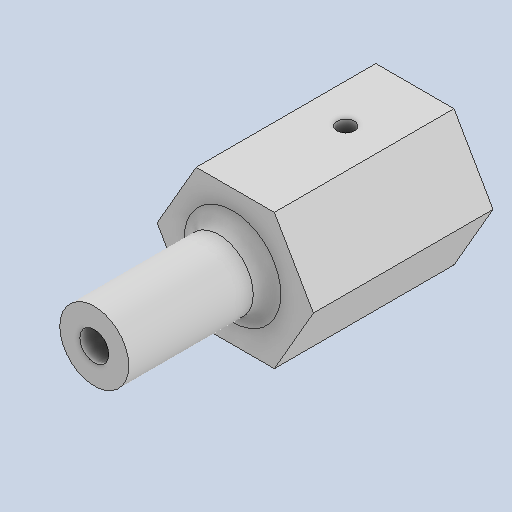
# Autodesk Inventor part: Acople_Motor
Saved by Autodesk Inventor 2022 (Build 260153000, 153)
## iProperties
Created: 2022-02-22
Part Number: Acople_Motor
Material: Generic
Document SubType Name: Modeling
Designer: katha
Density: 1 g/cm^3
Appearance: Default
Author: katha
Autodesk Inventor part; units mm, degrees
ref_plane "YZ Plane" through (0, 0, 0) normal (1, 0, 0) x (0, 1, 0)
ref_plane "XZ Plane" through (0, 0, 0) normal (0, 1, 0) x (-1, 0, 0)
ref_plane "XY Plane" through (0, 0, 0) normal (0, 0, 1) x (1, 0, 0)
sketch "Sketch1" plane through (0, 0, 0) normal (0, 0, 1) x (1, 0, 0)
  line L0 (-1.6732, 2.8981) -> (1.6732, 2.8981) projected
  line L1 (-3.3464, 0) -> (-1.6732, 2.8981) projected
  line L2 (-1.6732, -2.8981) -> (-3.3464, 0) projected
  line L3 (1.6732, -2.8981) -> (-1.6732, -2.8981) projected
  line L4 (3.3464, 0) -> (1.6732, -2.8981) projected
  line L5 (1.6732, 2.8981) -> (3.3464, 0) projected
  line L6 (3.0288, 4.8981) -> (5.8567, 0) projected
  line L7 (-2.627, 4.8981) -> (3.0288, 4.8981) projected
  line L8 (-5.4549, 0) -> (-2.627, 4.8981) projected
  line L9 (-2.627, -4.8981) -> (-5.4549, 0) projected
  line L10 (3.0288, -4.8981) -> (-2.627, -4.8981) projected
  line L11 (5.8567, 0) -> (3.0288, -4.8981) projected
  point P0 (0, 0)
extrude "Extrusion1" add sketch "Sketch1" against normal blind 10
sketch "Sketch2" plane through (0, 0, 0) normal (0, 0, 1) x (1, 0, 0)
  line L0 (3.0288, 4.8981) -> (-2.627, 4.8981) projected
  line L1 (-2.627, 4.8981) -> (-5.4549, 0) projected
  line L2 (-5.4549, 0) -> (-2.627, -4.8981) projected
  line L3 (-2.627, -4.8981) -> (3.0288, -4.8981) projected
  line L4 (3.0288, -4.8981) -> (5.8567, 0) projected
  line L5 (5.8567, 0) -> (3.0288, 4.8981) projected
  point P0 (0, 0)
extrude "Extrusion2" add sketch "Sketch2" along normal blind 3
sketch "Sketch3" plane through (0, 0, 3) normal (0, 0, 1) x (1, 0, 0)
  circle A0 centre (0, 0) radius 2.5
  circle A1 centre (0, 0) radius 1.05
  dimension "d4" = 5
  dimension "d5" = 2.1
  constraints: 2 centre point, 2 coincident
  measures "d4" diameter of A0
  measures "d5" diameter of A1
extrude "Extrusion3" add sketch "Sketch3" along normal blind 10
fillet "Fillet1" radius 1 1 edges at (-2.5, 0, 3)
sketch "Sketch4" plane through (-2.627, 4.8981, -10) normal (0, 1, 0) x (1, 0, 0)
  line L0 (5.6558, 0) -> (5.6558, -13) projected
  line L1 (0, 0) -> (5.6558, 0) projected
  line L2 (0, -13) -> (0, 0) projected
  line L3 (5.6558, -13) -> (0, -13) projected
  line L4 (0.9538, -10) -> (4.3002, -10) projected
  line L5 (5.6558, 0) -> (0, 0) projected
  line L6 (2.8279, 0) -> (2.8279, -10) construction
  circle A0 centre (2.8279, -5.002) radius 0.625
  point P0 (2.627, -10)
  point P1 (2.8279, 0)
  dimension "d9" = 1.25
  constraints: 1 centre point, 1 horizontal, 1 midpoint, 4 other
  measures "d9" diameter of A0
extrude "Extrusion4" cut sketch "Sketch4" against normal blind 10 contours A0
body "Solid1"
